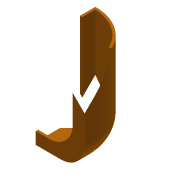
# Autodesk Inventor part: P_hips03_001
Saved by Autodesk Inventor 2016 (Build 200138000, 138)
## iProperties
Created: 2016-02-26
Part Number: P_hips03_001
Material: PC/ABS Plastic
Document SubType Name: Modeling
Designer: Mateusz
Density: 0.357273 g/cm^3
Appearance: Orange
Author: Mateusz
Autodesk Inventor part; units mm, degrees
sketch "Sketch1" plane through (0, 0, 0) normal (0, 0, 1) x (1, 0, 0)
  line L0 (0, 2) -> (37.5, 2) projected
  line L1 (-1, 52) -> (-1, 2) projected
  line L2 (-1, 52) -> (-1, 2)
  line L3 (-1, 2) -> (37.5, 2)
  line L4 (35.5, 4) -> (-1, 4)
  line L5 (1, 46.4068) -> (1, 39)
  line L6 (1, 39) -> (-1, 39)
  arc A0 (37.5, 13.5) -> (-1, 52) centre (-1, 13.5) ccw
  arc A1 (35.5, 13.5) -> (1, 49.9452) centre (-1, 13.5) ccw
  line L7 (37.5, 2) -> (37.5, 13.5)
  line L8 (35.5, 4) -> (35.5, 13.5)
  line L9 (1, 46.4068) -> (1, 49.9452)
  point P0 (0, 0)
  dimension "d1" = 2
  dimension "d2" = 2
  dimension "d3" = 13
  dimension "d6" = 2
  constraints: 16 end point, 5 vertical, 4 point on circle, 3 perpendicular, 3 point on line, 2 centre point, 2 tangent, 1 coincident
  measures "d1" distance between parallel lines of L0 L4
  measures "d2" distance between parallel lines of L1 L5
  measures "d3" distance from line of L1.start L6
  measures "d6" radial gap between concentric circles of A0 A1
ref_plane "Work Plane1" through (0, 0, 70) normal (0, 0, 1) x (1, 0, 0)
ref_plane "Work Plane2" through (0, 0, -70) normal (0, 0, -1) x (0, 1, 0)
ref_plane "Work Plane3" through (0, 0, -70) normal (0, 0, -1) x (0, 1, 0)
ref_plane "Work Plane4" through (0, 0, -75) normal (0, 0, -1) x (0, 1, 0)
extrude "Extrusion2" add sketch "Sketch1" against normal up to surface (75 mm away) contours L3 L1 L4 L8 A1 L9 L5 L6 A0 L7 L0
sketch "Sketch2" plane through (37.5, 2, -75) normal (0, 0, -1) x (-1, 0, 0)
  arc A0 (38.5, 50) -> (0, 11.5) centre (38.5, 11.5) ccw projected
  line L0 (0, 0) -> (0, 11.5) projected
  line L1 (38.5, 0) -> (0, 0) projected
  line L2 (0, 0) -> (38.5, 0)
  line L3 (38.5, 0) -> (38.5, 50)
  line L4 (38.5, 2) -> (38.5, 0) projected
  point P0 (37.5, -2)
  constraints: 4 end point, 1 collinear, 1 horizontal, 1 point on circle
extrude "Extrusion3" add sketch "Sketch2" against normal blind 2
sketch "Sketch3" plane through (-1, 4, 0) normal (0, 1, 0) x (1, 0, 0)
  line L0 (36.5, 73) -> (0, 73) projected
  line L1 (0, 0) -> (0, 73) projected
  line L2 (36.5, 0) -> (0, 0) projected
  line L3 (36.5, 0) -> (36.5, 73) projected
  line L4 (0, 0) -> (0, 73) projected
  line L5 (0, 65) -> (28.5, 65)
  line L6 (28.5, 65) -> (28.5, 0)
  line L7 (36.5, 0) -> (0, 0) projected
  line L8 (36.5, 0) -> (36.5, 73) projected
  point P0 (1, 0)
  dimension "d11" = 8
  dimension "d12" = 8
  constraints: 4 end point, 2 parallel, 2 point on line, 1 horizontal, 1 perpendicular
  measures "d11" distance between parallel lines of L3 L6
  measures "d12" distance between parallel lines of L0 L5
extrude "Extrusion4" cut sketch "Sketch3" against normal up to next contours L5 L6 L2 L1
fillet "Fillet1" radius 20 5 edges at (27.5, 3, -65) (35.5, 8.75, -73) (25.5071, 38.5923, -73) (37.5, 7.75, -75) (26.2236, 40.7236, -75)
body "Solid2"
